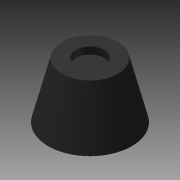
# Autodesk Inventor part: doorstop
Saved by Autodesk Inventor 2011 SP1 (Build 150282100, 282)
## iProperties
Created: 2012-01-18
Part Number: doorstop
Document SubType Name: Modeling
Designer: Christopher
Density: 1 g/cm^3
Author: Christopher
Autodesk Inventor part; units mm, degrees
ref_plane "YZ Plane" through (0, 0, 0) normal (1, 0, 0) x (0, 1, 0)
ref_plane "XZ Plane" through (0, 0, 0) normal (0, 1, 0) x (-1, 0, 0)
ref_plane "XY Plane" through (0, 0, 0) normal (0, 0, 1) x (1, 0, 0)
sketch "Sketch1" plane through (0, 0, 0) normal (0, 0, 1) x (1, 0, 0)
  line L0 (0, 0) -> (9.525, 0)
  line L1 (9.525, 0) -> (6.35, 12.7)
  line L2 (6.35, 12.7) -> (3.175, 12.7)
  line L3 (3.175, 12.7) -> (3.175, 11.1125)
  line L4 (3.175, 11.1125) -> (0, 11.1125)
  line L5 (0, 11.1125) -> (0, 0)
  dimension "d0" = 9.525
  dimension "d3" = 3.175
  dimension "d4" = 1.5875
  dimension "d5" = 11.1125
  constraints: 12 end point, 3 parallel, 1 horizontal, 1 perpendicular
  measures "d0" distance of L0.start L0.end
  measures "d3" distance of L3.end L4.end
  measures "d4" distance of L2.end L3.end
  measures "d5" distance of L4.end L0.start
revolve "Revolution1" add sketch "Sketch1" angle 360 about axis through (0, 11.1125, 0) along (0, -1, 0)
body "Solid1"
